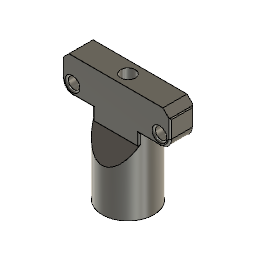
10.SensorMount) PLA Base Shaker Attachment (Autodesk Fusion 360 design; units mm, degrees)
Autodesk Fusion 360 part; units mm, degrees
ref_plane "WorkPlane1" through (0, 0, 0) normal (0, 0, 1) x (1, 0, 0)
sketch "Sketch1" plane through (0, 0, 0) normal (0, 0, 1) x (1, 0, 0)
  circle A0 centre (0, 0) radius 5.2
  circle A1 centre (0, 0) radius 7.5
  circle A2 centre (0, 0) radius 2.1
  dimension "d2" = 10.4
  dimension "d3" = 15
  dimension "d4" = 4.2
  constraint coincident A0.centre A1.centre
  measures "d2" diameter of A0
  measures "d3" diameter of A1
  measures "d4" diameter of A2
extrude "Extrude1" add sketch "Sketch1" along normal blind 20 contours A0 | A1
ref_plane "WorkPlane2" through (0, 0, 20) normal (0, 0, 1) x (1, 0, 0)
sketch "Sketch2" plane through (0, 0, 20) normal (0, 0, 1) x (1, 0, 0)
  circle A0 centre (0, 0) radius 7.5
extrude "Extrude2" add sketch "Sketch2" along normal blind 10 draft -22
extrude "Extrude3" cut 1 faces at (0.5514, -0.0339, 20) along direction (0, 0, 1) up to surface (10 mm away)
extrude "Extrude4" add sketch "Sketch1" against normal blind 1.6 contours A1
ref_plane "WorkPlane3" through (0, -3.5, 0) normal (0, 1, 0) x (0, 0, 1)
sketch "Sketch3" plane through (0, -3.5, 0) normal (0, 1, 0) x (1, 0, 0)
  line L0 (0, -16.8) -> (0, 0)
  line L1 (12.6, -25.9) -> (6.1, -25.9)
  line L2 (6, -19.9) -> (6, -16.8)
  line L3 (12.6, -25.9) -> (12.6, -19.9)
  line L4 (12.6, -22.9) -> (0, -22.9)
  line L5 (6.1, -29) -> (0, -29)
  circle A0 centre (12.6, -22.9) radius 3
  line L6 (6.1, -29) -> (6.1, -25.9)
  line L7 (12.6, -19.9) -> (6, -19.9)
  line L8 (6, -16.8) -> (0, -16.8)
  line L9 (0, -22.9) -> (15.6, -22.9)
  line L10 (0, -16.8) -> (0, -29)
  circle A1 centre (12.6, -22.9) radius 1.65
  line L11 (0, -1.5459) -> (0, -23.0712)
  line L12 (-6, -19.9) -> (-6, -16.8)
  line L13 (-6, -16.8) -> (0, -16.8)
  line L14 (-12.6, -19.9) -> (-6, -19.9)
  circle A2 centre (-12.6, -22.9) radius 3
  line L15 (-12.6, -25.9) -> (-6.1, -25.9)
  line L16 (-6.1, -29) -> (-6.1, -25.9)
  line L17 (-6.1, -29) -> (0, -29)
  circle A3 centre (-12.6, -22.9) radius 1.65
  line L18 (-6.1, -29) -> (6.1, -29)
  line L19 (-15.6, -22.9) -> (15.6, -22.9)
  line L20 (15.6, -22.9) -> (15.6, -30)
  line L21 (15.6, -30) -> (-15.6, -30)
  line L22 (-15.6, -30) -> (-15.6, -22.9)
  line L23 (3.4597, -30) -> (-3.4597, -30)
  dimension "d15" = 3.3
  dimension "d16" = 6.5
  dimension "d17" = 6
  dimension "d18" = 6
  dimension "d19" = 6.1
  dimension "d20" = 6
  dimension "d21" = 16.8
  dimension "d22" = 3.1
  dimension "d23" = 3.1
  dimension "d24" = 15.6
  constraint concentric A0 A1
  constraint vertical L2
  constraint horizontal L7
  constraint horizontal L4
  constraint vertical L0
  constraint parallel L1 L7
  constraint coincident L1.end L6
  constraint coincident L2.start L7
  constraint perpendicular L3 L7
  constraint perpendicular L2 L8
  constraint perpendicular L8 L10
  constraint coincident L5.end L10
  constraint perpendicular L5 L10
  constraint coincident L2.start L7.end
  constraint coincident L4.start L3
  constraint midpoint L4.start L3
  constraint coincident L4.end L10
  constraint coincident L4.start A0.centre
  constraint perpendicular L1 L6
  constraint horizontal L9
  constraint vertical L11
  constraint symmetric L1.end L11 L15.end
  constraint symmetric L0.start L11 L8.end
  constraint symmetric L5.start L11 L16.start
  constraint symmetric L2.start L11 L12.start
  constraint symmetric L2.end L11 L12.end
  constraint symmetric L5.end L11 L10.end
  constraint symmetric L1.start L11 L15.start
  constraint symmetric L3.end L11 L14.start
  constraint symmetric A0 L11 A2
  constraint symmetric A1 L11 A3
  constraint coincident L11.start L0
  constraint coincident L0.end origin
  constraint horizontal L18
  constraint coincident L5.start L6.start
  constraint horizontal L19
  constraint vertical L20
  constraint horizontal L21
  constraint vertical L22
  constraint coincident A2 L19.start
  constraint coincident L21 L23.end
  constraint coincident A2.centre L19
  constraint coincident L9.end L20
  measures "d15" diameter of A1
  measures "d16" distance of L1.end L1.start
  measures "d17" distance of L1.start L3.end
  measures "d18" diameter of A0
  measures "d19" distance of L5.start L5.end
  measures "d20" distance of L0.start L2.end
  measures "d21" distance of L0.start L0.end
  measures "d22" distance of L2.start L2.end
  measures "d23" distance of L1.end L5.start
  measures "d24" distance of L4.end L9.end
extrude "Extrude5" cut sketch "Sketch3" against normal blind 7 contours L1 L5 A0 L6 A2 L15 L16 L17 L18 L20 L21 L22 L23 | L1 L4 L5 A0 L6 L9 L10 L11 L18 L19 | L2 L4 A0 L7 L8 L9 L10 L11 L19 | L10 L11 L12 L13 L14 A2 L19 | L10 L11 A2 L15 L16 L17 L18 L19
extrude "Extrude6" add sketch "Sketch3" along normal blind 7 contours L1 L5 A0 L6 A2 L15 L16 L17 L18 L20 L21 L22 L23 | L3 L4 A0 L9 A1 L19 | L3 A0 L9 A1 L19 | L1 L4 L5 A0 L6 L9 L10 L11 L18 L19 | L3 A0 L9 A1 L19 | L3 L4 A0 L9 A1 L19 | L2 L4 A0 L7 L8 L9 L10 L11 L19 | L10 L11 L12 L13 L14 A2 L19 | L10 L11 A2 L15 L16 L17 L18 L19 | A2 A3 L19 | A2 A3 L19
ref_plane "WorkPlane4" through (0, 0, 30) normal (0, 0, 1) x (1, 0, 0)
sketch "Sketch4" plane through (0, 0, 30) normal (0, 0, 1) x (1, 0, 0)
  circle A0 centre (0, 0) radius 2.1
extrude "Extrude7" cut sketch "Sketch4" against normal up to surface (13.2 mm away)
ref_plane "WorkPlane5" through (-9, -4, 18.35) normal (1, 0, 0) x (0, 0, 1)
sketch "Sketch5" plane through (-9, 0, 0) normal (1, 0, 0) x (0, 1, 0)
  line L0 (-4.5, 19.9) -> (-4.5, 16.8)
  line L1 (-7.5, 16.8) -> (-4.5, 16.8)
  line L2 (-4.5, 16.8) -> (-4.5, 19.9)
  line L3 (7.5, 20) -> (3.5, 20)
  line L4 (-7.5, -1.6) -> (7.5, -1.6)
  line L5 (-3.5, 19.9) -> (-3.5, 16.8)
  line L6 (-3.5, 16.8) -> (-7.5, 10.8)
  line L7 (-4.5, 19.9) -> (-4.5, 19.9)
  line L8 (-4.5, 19.9) -> (-3.5, 19.9)
  line L9 (-3.5, 19.9) -> (3.5, 19.9)
  line L10 (-4.5, 19.9) -> (-3.5, 19.9)
  line L11 (-4.5, 19.9) -> (-3.5, 19.9)
  line L12 (-3.5, 19.9) -> (3.5, 19.9)
  line L13 (3.5, 19.9) -> (3.5, 20)
  line L14 (3.5, 20) -> (3.5, 19.9)
  line L15 (-7.5, 16.8) -> (-7.5, -1.6)
  point P0 (-3.5, 19.9)
  point P1 (-3.5, 16.8)
  dimension "d42" = 6
  constraint coincident P0 L5.start
  constraint coincident P1 L5.end
  constraint coincident L0.start L2.end
  constraint perpendicular L3 L7
  constraint perpendicular L5 L8
  constraint coincident L1.start L15.start
  constraint coincident L4.start L15.end
  constraint coincident L6.end L15
  measures "d42" distance of L6.end L1.start
extrude "Extrude8" cut sketch "Sketch5" along normal blind 17
chamfer "Chamfer1" distance 2 angle 45 2 edges at (15.6, 0, 30) (-15.6, 0, 30)
fillet "Fillet1" radius 0.5 18 edges at (-14.1383, -3.5, 22.3033) (11.0617, -3.5, 22.3033) (6.6332, -3.5, 18.35) (-15.6, -3.5, 25.45) (-14.7213, -3.5, 20.7787) (-9.6166, -3.5, 19.9) (9.6166, -3.5, 19.9) (14.7213, -3.5, 20.7787) (15.6, -3.5, 25.45) (-6.6332, -3.5, 18.35) (-9.6166, 3.5, 19.9) (-14.7213, 3.5, 20.7787) (-15.6, 3.5, 25.45) (15.6, 3.5, 25.45) (14.7213, 3.5, 20.7787) (9.6166, 3.5, 19.9) (15.6, 0, 28) (-15.6, 0, 28)
named bodies: "Bass Shaker 50mm M4 Bolt Adapter (With sensor)"
